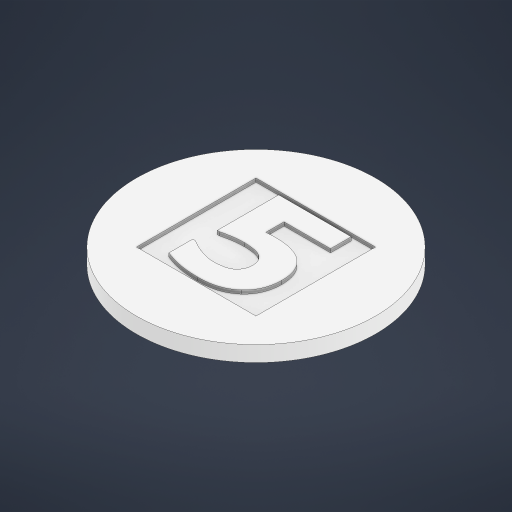
# Autodesk Inventor part: TopMarker1
Saved by Autodesk Inventor 2023.2 (Build 272271030, 271C)
## iProperties
Created: 2023-03-04
Part Number: TopMarker1
Material: Generic
Document SubType Name: Modeling
Designer: Elias Braun
Density: 1 g/cm^3
Appearance: Default
Author: Elias Braun
Autodesk Inventor part; units mm, degrees
ref_plane "YZ Plane" through (0, 0, 0) normal (1, 0, 0) x (0, 1, 0)
ref_plane "XZ Plane" through (0, 0, 0) normal (0, 1, 0) x (-1, 0, 0)
ref_plane "XY Plane" through (0, 0, 0) normal (0, 0, 1) x (1, 0, 0)
sketch "Sketch1" plane through (0, 0, 0) normal (0, 1, 0) x (-1, 0, 0)
  circle A0 centre (0, 0) radius 20
  dimension "d0" = 40
  constraints: 1 centre point, 1 coincident
  measures "d0" diameter of A0
extrude "Extrusion1" add sketch "Sketch1" along normal blind 2.6
sketch "Sketch2" plane through (0, 2.6, 0) normal (0, 1, 0) x (1, 0, 0)
  line L0 (10, -10) -> (-10, -10)
  line L1 (-10, -10) -> (-10, 10)
  line L2 (-10, 10) -> (10, 10)
  line L3 (10, 10) -> (10, -10)
  line L4 (10, -10) -> (-10, 10) construction
  line L5 (-10, -10) -> (10, 10) construction
  point P0 (0, 0)
  dimension "d3" = 20
  dimension "d4" = 20
  constraints: 12 end point, 2 midpoint, 2 parallel, 1 horizontal, 1 perpendicular
  measures "d3" distance of L0.start L0.end
  measures "d4" distance of L0.end L1.end
extrude "Extrusion2" cut sketch "Sketch2" against normal blind 0.6
sketch "Sketch4" plane through (0, 2, 0) normal (0, 1, 0) x (1, 0, 0)
  line L0 (-7.9065, 9.4518) -> (8.1246, 9.4518) construction
  line L1 (8.1246, 9.4518) -> (8.1246, -9.2337) construction
  line L2 (8.1246, -9.2337) -> (-7.9065, -9.2337) construction
  line L3 (-7.9065, -9.2337) -> (-7.9065, 9.4518) construction
  spline S0 degree 2 poles (6.9827, -2.6493) (6.9827, -4.0878) (6.0039, -6.5199) (5.04, -7.3948) knots 0 0 0 1 2 2 2
  spline S1 degree 2 poles (5.04, -7.3948) (4.076, -8.2698) (1.4363, -9.2337) (-0.4915, -9.2337) knots 0 0 0 1 2 2 2
  spline S2 degree 2 poles (-0.4915, -9.2337) (-2.5381, -9.2189) (-5.4744, -8.5516) (-6.4383, -8.1215) knots 0 0 0 1 2 2 2
  line L4 (-6.4383, -8.1215) -> (-6.4383, -4.1323)
  line L5 (-6.4383, -4.1323) -> (-6.0231, -4.1323)
  spline S3 degree 2 poles (-6.0231, -4.1323) (-5.6672, -4.3251) (-4.807, -4.8293) (-4.11, -5.0962) knots 0 0 0 1 2 2 2
  spline S4 degree 2 poles (-4.11, -5.0962) (-3.4575, -5.3483) (-2.108, -5.6894) (-1.2924, -5.6894) knots 0 0 0 1 2 2 2
  spline S5 degree 2 poles (-1.2924, -5.6894) (-0.5805, -5.6894) (1.0804, -5.3335) (1.5846, -4.8589) knots 0 0 0 1 2 2 2
  spline S6 degree 2 poles (1.5846, -4.8589) (1.9554, -4.4882) (2.3706, -3.5836) (2.3706, -2.8272) knots 0 0 0 1 2 2 2
  spline S7 degree 2 poles (2.3706, -2.8272) (2.3706, -2.1747) (1.8367, -1.2553) (1.4067, -0.9735) knots 0 0 0 1 2 2 2
  spline S8 degree 2 poles (1.4067, -0.9735) (0.7838, -0.5583) (-0.9958, -0.321) (-1.6334, -0.321) knots 0 0 0 1 2 2 2
  spline S9 degree 2 poles (-1.6334, -0.321) (-2.6419, -0.321) (-4.5549, -0.6473) (-5.2519, -0.8252) knots 0 0 0 1 2 2 2
  line L6 (-5.2519, -0.8252) -> (-5.6523, -0.8252)
  line L7 (-5.6523, -0.8252) -> (-5.6523, 9.4518)
  line L8 (-5.6523, 9.4518) -> (6.4785, 9.4518)
  line L9 (6.4785, 9.4518) -> (6.4785, 5.9965)
  line L10 (6.4785, 5.9965) -> (-1.3072, 5.9965)
  line L11 (-1.3072, 5.9965) -> (-1.3072, 2.9564)
  spline S10 degree 2 poles (-1.3072, 2.9564) (-0.9364, 2.986) (0.0868, 3.0157) (0.3686, 3.0157) knots 0 0 0 1 2 2 2
  spline S11 degree 2 poles (0.3686, 3.0157) (1.6884, 3.0157) (3.9129, 2.4818) (4.7879, 1.9331) knots 0 0 0 1 2 2 2
  spline S12 degree 2 poles (4.7879, 1.9331) (5.826, 1.251) (6.9827, -1.018) (6.9827, -2.6493) knots 0 0 0 1 2 2 2
  point P0 (0, 0)
  constraints: 2 other
extrude "Extrusion4" add sketch "Sketch4" along normal blind 0.6
body "Solid1"
